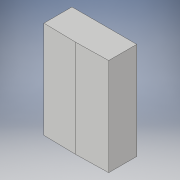
# Autodesk Inventor part: UWO-BLT-SS20-Test7
Saved by Autodesk Inventor 2017 (Build 210142000, 142)
## iProperties
Created: 2018-12-06
Part Number: UWO-BLT-SS20-Test7
Material: Generic
Document SubType Name: Modeling
Designer: mcgratta
Density: 1 g/cm^3
Appearance: Default
Author: mcgratta
Autodesk Inventor part; units mm, degrees
ref_plane "YZ Plane" through (0, 0, 0) normal (1, 0, 0) x (0, 1, 0)
ref_plane "XZ Plane" through (0, 0, 0) normal (0, 1, 0) x (-1, 0, 0)
ref_plane "XY Plane" through (0, 0, 0) normal (0, 0, 1) x (1, 0, 0)
sketch "Sketch1" plane through (0, 0, 0) normal (0, 1, 0) x (-1, 0, 0)
  line L0 (0, 0) -> (0, 39.624)
  line L1 (0, 39.624) -> (-45.72, 40.5765)
  line L2 (-45.72, 40.5765) -> (-91.44, 39.624)
  line L3 (-91.44, 39.624) -> (-91.44, 0)
  line L4 (-91.44, 0) -> (0, 0)
  dimension "d0" = 91.44
  dimension "d1" = 39.624
  dimension "d2" = 39.624
  dimension "d3" = 45.72
  dimension "d4" = 40.5765
  constraints: 10 end point, 1 parallel, 1 perpendicular, 1 vertical
  measures "d0" distance of L3.end L0.start
  measures "d1" distance of L2.end L3.end
  measures "d2" distance of L0.start L0.end
  measures "d3" distance from line of L1.end L3
  measures "d4" distance from line of L4 L1.end
extrude "Extrusion1" add sketch "Sketch1" along normal blind 137.16
body "Solid1"
